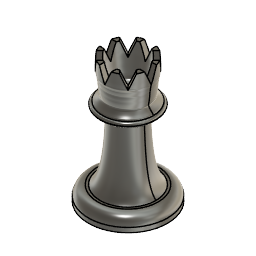
Regina (Autodesk Fusion 360 design; units mm, degrees)
part number: 2026-03-27-17-57-06-025
Autodesk Fusion 360 part; units mm, degrees
sketch "Regina" plane through (0, 0, 0) normal (0, 1, 0) x (1, 0, 0)
  line L0 (0, 0) -> (17, 0)
  line L1 (0, 0) -> (0, -41)
  line L2 (17, 0) -> (17, -2)
  line L3 (13, -6) -> (0, -6)
  line L4 (0, -41) -> (0, -39.2065) construction
  line L5 (3.0623, -35) -> (0, -35)
  line L6 (0, -35) -> (0, -39.2065)
  arc A0 (13, -6) -> (17, -2) centre (13, -2) ccw
  line L7 (0, -39) -> (0, -41)
  arc A1 (10.0008, -39) -> (10, -39) centre (10, -40) ccw
  line L8 (3.0623, -35) -> (10.9377, -35)
  line L9 (0, -37.1033) -> (10.9434, -37.1033)
  line L10 (11.9419, -36.0482) -> (11.9362, -35.945)
  arc A2 (10.9434, -37.1033) -> (11.9419, -36.0482) centre (10.9434, -36.1033) ccw
  arc A3 (11.9362, -35.945) -> (10.9377, -35) centre (10.9377, -36) ccw
  spline S0 degree 5 poles (0, -41) (0.2083, -40.9398) (0.6157, -40.8267) (1.1995, -40.6787) (1.9231, -40.5249) (2.7363, -40.4049) (3.4584, -40.3568) (4.0905, -40.3792) (4.6342, -40.4699) (5.0924, -40.6251) (5.4693, -40.8395) (5.7707, -41.1057) (6.0047, -41.4142) (6.1808, -41.7532) (6.3098, -42.1104) (6.403, -42.4744) (6.4712, -42.8361) (6.5241, -43.1902) (6.5701, -43.5357) (6.6153, -43.8747) (6.6643, -44.2102) (6.7194, -44.545) (6.7805, -44.8795) (6.8453, -45.2114) (6.9105, -45.5373) (6.9731, -45.8546) (7.0311, -46.1635) (7.085, -46.4688) (7.138, -46.7792) (7.1936, -47.1039) (7.2549, -47.4491) (7.3229, -47.8152) (7.3951, -48.1929) (7.4664, -48.5665) (7.531, -48.9193) (7.5841, -49.2385) (7.6231, -49.5189) (7.6499, -49.7696) (7.6697, -50.0089) (7.6883, -50.2559) (7.711, -50.5249) (7.7399, -50.8159) (7.7746, -51.1193) (7.8131, -51.4217) (7.8528, -51.7111) (7.8909, -51.9831) (7.9257, -52.2421) (7.9554, -52.4973) (7.9791, -52.7592) (7.9959, -53.0363) (8.0054, -53.3331) (8.007, -53.5884) (8.0048, -53.7902) (8.0019, -53.9293) (8, -54) knots 0 0 0 0 0 0 0.02 0.04 0.06 0.08 0.1 0.12 0.14 0.16 0.18 0.2 0.22 0.24 0.26 0.28 0.3 0.32 0.34 0.36 0.38 0.4 0.42 0.44 0.46 0.48 0.5 0.52 0.54 0.56 0.58 0.6 0.62 0.64 0.66 0.68 0.7 0.72 0.74 0.76 0.78 0.8 0.82 0.84 0.86 0.88 0.9 0.92 0.94 0.96 0.98 1 1 1 1 1 1
  line L11 (8, -54) -> (10, -54)
  spline S1 degree 5 poles (10, -54) (10.0003, -53.9643) (10.0009, -53.893) (10.0015, -53.7863) (10.0021, -53.6443) (10.0022, -53.4675) (10.0017, -53.2913) (10.0008, -53.1155) (9.9996, -52.94) (9.9984, -52.7646) (9.9975, -52.5889) (9.9973, -52.4126) (9.9978, -52.2353) (9.9993, -52.057) (10.0013, -51.8776) (10.0035, -51.6974) (10.0048, -51.5172) (10.0047, -51.3382) (10.003, -51.1625) (9.9998, -50.9932) (9.9971, -50.8349) (9.9962, -50.6912) (9.997, -50.5614) (9.999, -50.4427) (10.001, -50.3302) (10.0023, -50.218) (10.0027, -50.0997) (10.0018, -49.9699) (9.9999, -49.825) (9.9968, -49.6648) (9.9924, -49.4929) (9.9865, -49.3152) (9.9792, -49.1386) (9.971, -48.9695) (9.9624, -48.8122) (9.9548, -48.6674) (9.9498, -48.5327) (9.9485, -48.4043) (9.9508, -48.2781) (9.9552, -48.1515) (9.9578, -48.0242) (9.9542, -47.8975) (9.9404, -47.7728) (9.9147, -47.6506) (9.8786, -47.5297) (9.8367, -47.407) (9.7944, -47.2791) (9.7566, -47.1427) (9.7263, -46.9962) (9.7031, -46.8396) (9.685, -46.6745) (9.6688, -46.5033) (9.6514, -46.3293) (9.6302, -46.1561) (9.6043, -45.9872) (9.5742, -45.8253) (9.5412, -45.6726) (9.5073, -45.5295) (9.4745, -45.3949) (9.4447, -45.2651) (9.4194, -45.1349) (9.3997, -44.999) (9.3857, -44.8526) (9.3769, -44.6934) (9.3716, -44.522) (9.3676, -44.341) (9.3626, -44.1544) (9.3546, -43.9664) (9.3422, -43.781) (9.3251, -43.6008) (9.3045, -43.4266) (9.2819, -43.2581) (9.2593, -43.0941) (9.2383, -42.9328) (9.22, -42.7721) (9.2045, -42.6102) (9.1909, -42.4455) (9.1778, -42.2768) (9.1638, -42.1036) (9.1473, -41.9261) (9.1273, -41.7453) (9.1032, -41.5633) (9.0751, -41.3824) (9.0431, -41.2052) (9.0082, -41.0339) (8.9713, -40.8699) (8.934, -40.7138) (8.898, -40.5652) (8.8656, -40.4228) (8.8396, -40.2852) (8.8232, -40.1502) (8.8205, -40.016) (8.8353, -39.881) (8.8703, -39.7444) (8.9259, -39.607) (8.9989, -39.4716) (9.0821, -39.3435) (9.1671, -39.2279) (9.2462, -39.1285) (9.3149, -39.0458) (9.3748, -38.9745) (9.4331, -38.9045) (9.4986, -38.825) (9.5792, -38.7278) (9.6773, -38.6117) (9.7913, -38.4807) (9.9167, -38.342) (10.0475, -38.2039) (10.1775, -38.0737) (10.302, -37.9554) (10.4179, -37.8484) (10.5238, -37.7498) (10.6193, -37.655) (10.7045, -37.5589) (10.7796, -37.4576) (10.8449, -37.3489) (10.8892, -37.2551) (10.918, -37.1808) (10.9352, -37.1294) (10.9434, -37.1033) knots 0 0 0 0 0 0 0.00869565 0.0173913 0.02608696 0.03478261 0.04347826 0.05217391 0.06086957 0.06956522 0.07826087 0.08695652 0.09565217 0.10434783 0.11304348 0.12173913 0.13043478 0.13913043 0.14782609 0.15652174 0.16521739 0.17391304 0.1826087 0.19130435 0.2 0.20869565 0.2173913 0.22608696 0.23478261 0.24347826 0.25217391 0.26086957 0.26956522 0.27826087 0.28695652 0.29565217 0.30434783 0.31304348 0.32173913 0.33043478 0.33913043 0.34782609 0.35652174 0.36521739 0.37391304 0.3826087 0.39130435 0.4 0.40869565 0.4173913 0.42608696 0.43478261 0.44347826 0.45217391 0.46086957 0.46956522 0.47826087 0.48695652 0.49565217 0.50434783 0.51304348 0.52173913 0.53043478 0.53913043 0.54782609 0.55652174 0.56521739 0.57391304 0.5826087 0.59130435 0.6 0.60869565 0.6173913 0.62608696 0.63478261 0.64347826 0.65217391 0.66086957 0.66956522 0.67826087 0.68695652 0.69565217 0.70434783 0.71304348 0.72173913 0.73043478 0.73913043 0.74782609 0.75652174 0.76521739 0.77391304 0.7826087 0.79130435 0.8 0.80869565 0.8173913 0.82608696 0.83478261 0.84347826 0.85217391 0.86086957 0.86956522 0.87826087 0.88695652 0.89565217 0.90434783 0.91304348 0.92173913 0.93043478 0.93913043 0.94782609 0.95652174 0.96521739 0.97391304 0.9826087 0.99130435 1 1 1 1 1 1
  line L12 (10.0315, -52.8303) -> (9.9685, -49.1697)
  line L13 (-1.0096, -55) -> (-3, -55) construction
  line L14 (-3, -55) -> (-1.0096, -55) construction
  line L15 (-3, -55) -> (3, -55)
  line L16 (-3, -55) -> (0, -48)
  line L17 (0, -48) -> (3, -55)
  spline S2 degree 5 poles (7, -35) (7.0241, -33.463) (7.0927, -30.4328) (7.257, -26.0189) (7.6072, -20.4148) (8.3706, -14.1076) (9.4058, -9.9718) (10.541, -7.6389) (11.4828, -6.4802) (12, -6) knots 0 0 0 0 0 0 0.2 0.4 0.6 0.8 1 1 1 1 1 1
  line L18 (10.7838, -7.1292) -> (13.2162, -4.8708)
  point P0 (5.6353, -41)
  point P1 (6.4544, -42.7608)
  point P2 (6.7049, -44.4511)
  point P3 (7, -46)
  point P4 (7.2683, -47.5188)
  point P5 (7.5908, -49.2968)
  point P6 (7.6929, -50.3049)
  point P7 (7.8324, -51.5607)
  point P8 (7.9675, -52.6412)
  point P9 (10, -53)
  point P10 (10, -52)
  point P11 (10, -51)
  point P12 (10, -50.3822)
  point P13 (10, -49.8453)
  point P14 (9.9685, -48.9259)
  point P15 (9.951, -48.2884)
  point P16 (9.9322, -47.743)
  point P17 (9.7687, -47.1812)
  point P18 (9.6508, -46.3325)
  point P19 (9.5, -45.5)
  point P20 (9.3886, -44.8701)
  point P21 (9.3475, -43.8691)
  point P22 (9.2378, -42.9231)
  point P23 (9.1555, -42.0181)
  point P24 (9, -41)
  point P25 (8.8377, -40.2561)
  point P26 (8.9191, -39.6317)
  point P27 (9.2788, -39.0895)
  point P28 (9.5164, -38.8037)
  point P29 (10.1272, -38.125)
  point P30 (10.6702, -37.5956)
  dimension "d1" = 17
  dimension "d4" = 4
  dimension "d7" = 1
  constraint coincident L0.start L1.start
  constraint horizontal L0
  constraint perpendicular L0 L1
  constraint perpendicular L0 L2
  constraint coincident L1 L3.end
  constraint perpendicular L1 L3
  constraint coincident L1 L4.end
  constraint horizontal L5
  constraint vertical L6
  constraint tangent L2 A0
  constraint tangent L3 A0
  constraint vertical L7
  constraint parallel L5 L8
  constraint midpoint L6 L9.start
  constraint perpendicular L1 L9
  constraint tangent L9 A2
  constraint tangent L10 A2
  constraint tangent L8 A3
  constraint tangent L10 A3
  constraint equal A2 A3
  constraint horizontal L11
  constraint midpoint P11 L12
  constraint horizontal L13
  constraint parallel L14 L15
  constraint midpoint L8 S2.start
  constraint coincident L3 S2.end
  constraint midpoint S2.end L18
  measures "d1" distance of L0.start L0.end
  measures "d4" radius of A0
  measures "d7" radius of A2
revolve "Revolve2" add sketch "Regina" angle 360 about axis through (0, 0, 0) along (0, 0, 1) contours L0 L1 L2 L3 A0 | L1 L3 L5 L8 S2 | L1 L5 L6 L8 L9 L10 A2 A3 | L1 L6 L7 L9 S0 L11 S1
extrude "Extrude3" cut sketch "Regina" along normal blind 14 contours L15 L16 L17
pattern_circular "C-Pattern3" count 8 over 360 about axis through (0, 0, 37.1033) along (0, 0, 1) of "Extrude3"
named bodies: "Regina"
